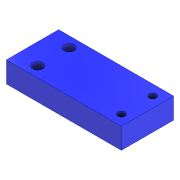
# Autodesk Inventor part: x_axis_extensor
Saved by Autodesk Inventor 2022 (Build 260153000, 153)
## iProperties
Created: 2021-08-05
Part Number: x_axis_extensor
Material: Generic
Document SubType Name: Modeling
Designer: nnico
Density: 1 g/cm^3
Appearance: Blue - Wall Paint - Glossy
Author: nnico
Autodesk Inventor part; units mm, degrees
ref_plane "YZ Plane" through (0, 0, 0) normal (1, 0, 0) x (0, 1, 0)
ref_plane "XZ Plane" through (0, 0, 0) normal (0, 1, 0) x (-1, 0, 0)
ref_plane "XY Plane" through (0, 0, 0) normal (0, 0, 1) x (1, 0, 0)
sketch "Sketch1" plane through (0, 0, 0) normal (0, 1, 0) x (-1, 0, 0)
  line L0 (50, -12.5) -> (-5, -12.5)
  line L1 (-5, -12.5) -> (-5, 12.5)
  line L2 (-5, 12.5) -> (50, 12.5)
  line L3 (50, 12.5) -> (50, -12.5)
  line L4 (50, 0) -> (-5, 0) construction
  line L5 (0, -12.5) -> (0, 12.5) construction
  circle A0 centre (0, -7.5) radius 1.75
  circle A1 centre (0, 7.5) radius 1.75
  line L6 (15, 12.5) -> (15, -12.5) construction
  point P0 (0, 0)
  point P1 (0, 0)
  dimension "d0" = 25
  dimension "d1" = 5
  dimension "d2" = 3.5
  dimension "d3" = 3.5
  dimension "d4" = 15
  dimension "d5" = 15
  dimension "d6" = 35
  constraints: 14 end point, 6 point on line, 3 midpoint, 3 perpendicular, 2 centre point, 2 parallel, 1 coincident, 1 horizontal, 1 symmetric about line
  measures "d0" distance of L0.end L1.end
  measures "d1" distance of L0.end L5.start
  measures "d2" diameter of A0
  measures "d3" diameter of A1
  measures "d4" distance of A1.centre A0.centre
  measures "d5" distance of L6.end L5.start
  measures "d6" distance of L2.end L6.start
extrude "Extrusion1" add sketch "Sketch1" along normal blind 10
sketch "Sketch2" plane through (0, 10, 0) normal (0, 1, 0) x (1, 0, 0)
  line L0 (-50, -12.5) -> (5, -12.5) construction
  line L1 (-40, -12.5) -> (-40, 12.5) construction
  line L2 (5, 12.5) -> (-50, 12.5) construction
  circle A0 centre (-40, 7.5) radius 2.5
  circle A1 centre (-40, -7.5) radius 2.5
  line L3 (-50, 12.5) -> (-50, -12.5) construction
  line L4 (-50, 0) -> (5, 0) construction
  line L5 (5, -12.5) -> (5, 12.5) construction
  point P0 (0, 0)
  dimension "d9" = 10
  dimension "d10" = 5
  dimension "d11" = 5
  dimension "d12" = 15
  constraints: 4 end point, 4 point on line, 2 centre point, 2 midpoint, 1 symmetric about line, 1 vertical
  measures "d9" distance of L2.end L1.end
  measures "d10" diameter of A0
  measures "d11" diameter of A1
  measures "d12" distance of A1.centre A0.centre
extrude "Extrusion2" cut sketch "Sketch2" against normal blind 6
body "Solid1"
